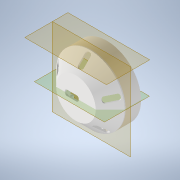
# Autodesk Inventor part: GehauseteilC
Saved by Autodesk Inventor 2020.2 (Build 242310000, 310)
## iProperties
Created: 2020-02-13
Part Number: GehauseteilC
Material: Generisch
Document SubType Name: Modeling
Designer: Max
Density: 1 g/cm^3
Appearance: Vorgabe
Author: Max
Autodesk Inventor part; units mm, degrees
ref_plane "YZ Plane" through (0, 0, 0) normal (1, 0, 0) x (0, 1, 0)
sketch "Skizze1" plane through (0, 0, 0) normal (0, 1, 0) x (-1, 0, 0)
  line L0 (0, 58.25) -> (0, 50.9382)
  line L1 (0, 85.6191) -> (0, -26.0665)
  line L2 (62.5, 0) -> (62.5, -3)
  line L3 (-64.5, 0) -> (64.5, 0) projected
  line L4 (0, 58.25) -> (-37.25, 58.25)
  line L5 (-37.25, 58.25) -> (-64.5, 31)
  line L6 (-64.5, 31) -> (-64.5, 0)
  line L7 (-64.5, 0) -> (-61.5, 0)
  line L8 (-61.5, 29.7574) -> (-36.0074, 55.25)
  line L9 (-36.0074, 55.25) -> (0, 55.25)
  line L10 (-61.5, 29.7574) -> (-61.5, 0)
  line L11 (0, 55.25) -> (0, 58.25)
  line L12 (64.5, 0) -> (-61.5, 0)
  point P0 (0, 0)
  point P1 (0, 0)
  point P2 (0, 55.25)
  dimension "d116" = 135
  dimension "d117" = 31
  dimension "d118" = 3
  dimension "d119" = 3
  dimension "d120" = 3
  dimension "d121" = 129
  dimension "d123" = 58.25
  constraints: 22 end point, 2 horizontal, 2 parallel, 2 perpendicular, 2 point on line, 1 collinear, 1 vertical, 5 other
  measures "d116" angle of L5 L6
  measures "d117" distance of L5.end L6.end
  measures "d118" distance between parallel lines of L6 L10
  measures "d119" distance between parallel lines of L5 L8
  measures "d120" distance between parallel lines of L4 L9
  measures "d121" diameter of L6 L1
  measures "d123" distance from line of point (0, 0) L4
revolve "Umdrehung1" add sketch "Skizze1" angle 360 about axis through (0, 0, 85.6191) along (0, 0, -1) contours L0 L9 L8 L10 L3 L6 L5 L4
ref_plane "Arbeitsebene12" through (0, 0, 29.125) normal (0, 0, 1) x (1, 0, 0)
ref_plane "Arbeitsebene16" through (-19.78, -4.15, 53.9382) normal (0, 0, 1) x (1, 0, 0)
ref_plane "Arbeitsebene13" through (-26.5595, -36.5552, 47.0027) normal (-0.4156269, -0.5720614, 0.7071068) x (-0.4156269, -0.5720614, -0.7071068)
sketch "Skizze26" plane through (-26.5595, -36.5552, 47.0027) normal (-0.4156269, -0.5720614, 0.7071068) x (-0.4156269, -0.5720614, -0.7071068)
  line L0 (-9, -4.15) -> (9, -4.15) projected
  line L1 (9, 4.15) -> (-9, 4.15) projected
  line L2 (12, -1.15) -> (12, 1.15) projected
  line L3 (-12, 1.15) -> (-12, -1.15) projected
  line L4 (5, -1.5) -> (5, 1.5) projected
  line L5 (5, 1.5) -> (9, 1.5) projected
  line L6 (9, 1.5) -> (9, -1.5) projected
  line L7 (9, -1.5) -> (5, -1.5) projected
  arc A0 (12, 1.15) -> (9, 4.15) centre (9, 1.15) ccw projected
  line L8 (9, 4.15) -> (-9, 4.15) projected
  arc A1 (-9, 4.15) -> (-12, 1.15) centre (-9, 1.15) ccw projected
  line L9 (-12, 1.15) -> (-12, -1.15) projected
  arc A2 (-12, -1.15) -> (-9, -4.15) centre (-9, -1.15) ccw projected
  line L10 (-9, -4.15) -> (9, -4.15) projected
  arc A3 (9, -4.15) -> (12, -1.15) centre (9, -1.15) ccw projected
  line L11 (12, -1.15) -> (12, 1.15) projected
  line L12 (14.0924, -1.5) -> (14.0924, 1.5) projected
  line L13 (14.0924, 1.5) -> (18.0924, 1.5) projected
  line L14 (18.0924, 1.5) -> (18.0924, -1.5) projected
  line L15 (18.0924, -1.5) -> (14.0924, -1.5) projected
  arc A4 (21.0924, 1.15) -> (18.0924, 4.15) centre (18.0924, 1.15) ccw projected
  line L16 (18.0924, 4.15) -> (0.0924, 4.15) projected
  arc A5 (0.0924, 4.15) -> (-2.9076, 1.15) centre (0.0924, 1.15) ccw projected
  line L17 (-2.9076, 1.15) -> (-2.9076, -1.15) projected
  arc A6 (-2.9076, -1.15) -> (0.0924, -4.15) centre (0.0924, -1.15) ccw projected
  line L18 (0.0924, -4.15) -> (18.0924, -4.15) projected
  arc A7 (18.0924, -4.15) -> (21.0924, -1.15) centre (18.0924, -1.15) ccw projected
  line L19 (21.0924, -1.15) -> (21.0924, 1.15) projected
  ellipse E0 centre (-20.635, 0.0005) end of major axis (-20.635, 64.5005) minor radius 45.6084 projected
  line L20 (0.0924, 5.15) -> (18.0924, 5.15)
  line L21 (22.0924, 1.15) -> (22.0924, -1.15)
  line L22 (18.0924, -5.15) -> (0.0924, -5.15)
  line L23 (-3.9076, -1.15) -> (-3.9076, 1.15)
  arc A8 (-3.9076, -1.15) -> (0.0924, -5.15) centre (0.0924, -1.15) ccw
  arc A9 (0.0924, 5.15) -> (-3.9076, 1.15) centre (0.0924, 1.15) ccw
  arc A10 (22.0924, 1.15) -> (18.0924, 5.15) centre (18.0924, 1.15) ccw
  arc A11 (18.0924, -5.15) -> (22.0924, -1.15) centre (18.0924, -1.15) ccw
  point P0 (1.2853, 0.0005)
  point P1 (-11.9204, -4.15)
  point P2 (12.2156, -4.15)
  point P3 (-6.7639, 0.85)
  point P4 (6.7639, 0.85)
  dimension "d124" = 1
  dimension "d125" = 1
  dimension "d126" = 1
  dimension "d127" = 1
  constraints: 10 point on circle, 8 end point, 4 centre point, 4 coincident, 4 tangent, 2 parallel, 2 point on line, 1 horizontal, 1 perpendicular, 1 other
  measures "d124" distance between parallel lines of L20 L16
  measures "d125" distance between parallel lines of L22 L18
  measures "d126" distance between parallel lines of L17 L23
  measures "d127" distance between parallel lines of L19 L21
extrude "Extrusion14" cut sketch "Skizze26" against normal mid plane 10 contours A6 L17 A5 L1 A0 L2 A3 L0 | L0 L18 A7 L19 A4 L16 L1 A9 L20 A10 L21 A11 L22 A8 | L0 A8 L23 A9 L1 A5 L17 A6 | A3 L2 A0 L16 A4 L19 A7 L18 | L4 L5 L6 L7 | L12 L13 L14 L15
ref_plane "Arbeitsebene14" through (-20.7407, -28.5463, 37.1032) normal (-0.4156269, -0.5720614, 0.7071068) x (-0.4156269, -0.5720614, -0.7071068)
ref_plane "Arbeitsebene15" through (0, 70, 0) normal (0, 1, 0) x (-1, 0, 0)
sketch "Skizze32" plane through (0, 70, 0) normal (0, 1, 0) x (-1, 0, 0)
  line L0 (-3.17, 8.66) -> (3.17, 8.66) projected
  line L1 (-3.17, 5.8) -> (3.17, 5.8) projected
  line L2 (-25.5797, 11.4942) -> (-36.763, 11.4942)
  line L3 (-36.763, 11.4942) -> (-36.763, -1.4577)
  line L4 (-36.763, -1.4577) -> (-25.5797, -1.4577)
  line L5 (-25.5797, -1.4577) -> (-25.5797, 11.4942)
  point P0 (0, 0)
  constraints: 8 end point, 2 parallel, 1 horizontal, 1 perpendicular
extrude "Kabelauslass" [suppressed]
pattern_circular "Runde Anordnung3" count 5 over 360 about axis through (0, 0, -10) along (0, 0, 1) of "Extrusion14"
ref_plane "Arbeitsebene17" through (-7.78, 0, 44.25) normal (0, 0, 1) x (0, -1, 0)
sketch "Skizze33" plane through (-7.78, 0, 44.25) normal (0, 0, 1) x (0, -1, 0)
  circle A0 centre (13.8, -12.5) radius 3
  circle A1 centre (13.8, 12.5) radius 3
  circle A2 centre (-13.8, 12.5) radius 3
  circle A3 centre (-13.8, -12.5) radius 3
  circle A4 centre (13.8, 12.5) radius 1.5 projected
  circle A5 centre (-13.8, 12.5) radius 1.5 projected
  circle A6 centre (13.8, -12.5) radius 1.5 projected
  circle A7 centre (-13.8, -12.5) radius 1.5 projected
  point P0 (0, 7.78)
  dimension "d131" = 6
  dimension "d132" = 6
  dimension "d133" = 6
  dimension "d134" = 6
  constraints: 4 centre point
  measures "d131" diameter of A1
  measures "d132" diameter of A0
  measures "d133" diameter of A3
  measures "d134" diameter of A2
extrude "Extrusion19" add sketch "Skizze33" along normal up to next
ref_plane "Arbeitsebene19" through (-41.4943, 13.4828, 32.5889) normal (-0.6724985, 0.218508, 0.7071068) x (0.309017, 0.9510565, 0)
sketch "Skizze35" plane through (-41.4943, 13.4828, 32.5889) normal (-0.6724985, 0.218508, 0.7071068) x (0.309017, 0.9510565, 0)
  circle A0 centre (13.8, -12.5) radius 1.5 projected
  circle A1 centre (13.8, 12.5) radius 1.5 projected
  circle A2 centre (-13.8, 12.5) radius 1.5 projected
  circle A3 centre (-13.8, -12.5) radius 1.5 projected
  circle A4 centre (13.8, -12.5) radius 3
  circle A5 centre (13.8, 12.5) radius 3
  circle A6 centre (-13.8, 12.5) radius 3
  circle A7 centre (-13.8, -12.5) radius 3
  point P0 (-0.0005, -7.8071)
  dimension "d143" = 6
  dimension "d144" = 6
  dimension "d145" = 6
  dimension "d146" = 6
  constraints: 4 centre point, 4 coincident
  measures "d143" diameter of A5
  measures "d144" diameter of A6
  measures "d145" diameter of A7
  measures "d146" diameter of A4
extrude "Extrusion20" add sketch "Skizze35" along normal up to next
sketch "Skizze36" plane through (-41.4943, 13.4828, 32.5889) normal (-0.6724985, 0.218508, 0.7071068) x (0.309017, 0.9510565, 0)
  line L0 (17.05, -17.5) -> (17.05, 17.5) projected
  line L1 (17.05, 17.5) -> (-17.05, 17.5) projected
  line L2 (-17.05, 17.5) -> (-17.05, -17.5) projected
  line L3 (-17.05, -17.5) -> (17.05, -17.5) projected
  line L4 (-15.55, -16) -> (-15.55, 16)
  line L5 (15.55, 16) -> (15.55, -16)
  line L6 (5.35, 17.5) -> (5.35, 16)
  line L7 (-5.35, 17.5) -> (-5.35, 16)
  line L8 (5.35, -17.5) -> (5.35, -16)
  line L9 (-5.35, -17.5) -> (-5.35, -16)
  line L10 (15.55, -16) -> (5.35, -16)
  line L11 (-5.35, -16) -> (-15.55, -16)
  line L12 (-15.55, 16) -> (-5.35, 16)
  line L13 (5.35, 16) -> (15.55, 16)
  line L14 (-17.05, -17.5) -> (-17.05, 17.5)
  line L15 (17.05, 17.5) -> (17.05, -17.5)
  line L16 (17.05, -17.5) -> (5.35, -17.5)
  line L17 (-5.35, -17.5) -> (-17.05, -17.5)
  line L18 (-17.05, 17.5) -> (-5.35, 17.5)
  line L19 (5.35, 17.5) -> (17.05, 17.5)
  point P0 (-0.0005, -7.8071)
  dimension "d147" = 1.5
  dimension "d149" = 1.5
  dimension "d151" = 10.7
  dimension "d152" = 11.7
  dimension "d153" = 10.7
  dimension "d154" = 11.7
  constraints: 32 end point, 12 perpendicular, 10 parallel, 4 horizontal, 4 point on line
  measures "d147" distance between parallel lines of L5 L0
  measures "d149" distance between parallel lines of L2 L4
  measures "d151" distance from line of L7 L6.end
  measures "d152" distance between parallel lines of L0 L6
  measures "d153" distance between parallel lines of L9 L8
  measures "d154" distance between parallel lines of L0 L8
extrude "Extrusion21" add sketch "Skizze36" along normal up to next contours L3 L8 L10 L5 L13 L6 L1 L0 | L3 L2 L1 L7 L12 L4 L11 L9
pattern_circular "Runde Anordnung4" count 5 over 360 about axis through (0, 0, 15.5) along (0, 0, -1) of "Extrusion20"
pattern_circular "Runde Anordnung5" count 5 over 360 about axis through (0, 0, 15.5) along (0, 0, -1) of "Extrusion21"
sketch "Skizze40" plane through (4.72, -13.8, 44.25) normal (0, 0, -1) x (-1, 0, 0)
  line L0 (-5, -3.25) -> (-5, 30.85) projected
  line L1 (30, -3.25) -> (-5, -3.25) projected
  line L2 (30, 30.85) -> (30, -3.25) projected
  line L3 (-5, 30.85) -> (30, 30.85) projected
  line L4 (-5, -3.25) -> (30, -3.25)
  line L5 (30, 30.85) -> (-5, 30.85)
  line L6 (-3.5, -1.75) -> (28.5, -1.75)
  line L7 (28.5, 29.35) -> (-3.5, 29.35)
  line L8 (28.5, 8.45) -> (30, 8.45)
  line L9 (28.5, 19.15) -> (30, 19.15)
  line L10 (-5, 8.45) -> (-3.5, 8.45)
  line L11 (-5, 19.15) -> (-3.5, 19.15)
  line L12 (-5, 30.85) -> (-5, 19.15)
  line L13 (-5, 8.45) -> (-5, -3.25)
  line L14 (-3.5, 29.35) -> (-3.5, 19.15)
  line L15 (-3.5, 8.45) -> (-3.5, -1.75)
  line L16 (28.5, -1.75) -> (28.5, 8.45)
  line L17 (28.5, 19.15) -> (28.5, 29.35)
  line L18 (30, -3.25) -> (30, 8.45)
  line L19 (30, 19.15) -> (30, 30.85)
  point P0 (4.72, 13.8)
  point P1 (30, 19.15)
  point P2 (-5, 19.15)
  dimension "d182" = 1.5
  dimension "d184" = 1.5
  dimension "d185" = 10.7
  dimension "d186" = 11.7
  dimension "d187" = 10.7
  dimension "d188" = 11.7
  constraints: 32 end point, 11 perpendicular, 10 parallel, 2 horizontal
  measures "d182" distance between parallel lines of L3 L7
  measures "d184" distance between parallel lines of L6 L1
  measures "d185" distance between parallel lines of L11 L10
  measures "d186" distance between parallel lines of L3 L11
  measures "d187" distance between parallel lines of L9 L8
  measures "d188" distance between parallel lines of L3 L9
extrude "Extrusion25" add sketch "Skizze40" against normal up to next contours L0 L10 L15 L6 L16 L8 L2 L1 | L0 L3 L2 L9 L17 L7 L14 L11
sketch "Skizze41" plane through (-7.78, 0, 44.25) normal (0, 0, -1) x (-1, 0, 0)
  line L0 (-17.5, -5.35) -> (-17.5, -17.05) projected
  line L1 (-17.5, 5.35) -> (-16, 5.35) projected
  line L2 (-17.5, -5.35) -> (-16, -5.35)
  line L3 (-16, -5.35) -> (-16, 5.35)
  line L4 (-16, 5.35) -> (-17.5, 5.35)
  line L5 (-17.5, 5.35) -> (-17.5, -5.35)
  line L6 (17.5, 17.05) -> (17.5, 5.35) projected
  line L7 (16, -5.35) -> (17.5, -5.35)
  line L8 (17.5, -5.35) -> (17.5, 5.35)
  line L9 (17.5, 5.35) -> (16, 5.35)
  line L10 (16, 5.35) -> (16, -5.35)
  point P0 (-7.78, 0)
  constraints: 16 end point, 4 parallel, 2 horizontal, 2 perpendicular
ref_plane "Arbeitsebene22" through (0.72, -5.3, 50.45) normal (0, 0, 1) x (1, 0, 0)
extrude "Extrusion26" add sketch "Skizze41" against normal up to surface (4.8 mm away) from surface at -6.2
sketch "Skizze42" plane through (-5.3495, 31.2555, 44.9633) normal (0, -0.7071068, -0.7071068) x (-1, 0, 0)
  line L0 (-10.7, 35) -> (-10.7, 33.5) projected
  line L1 (0, 35) -> (11.7, 35) projected
  line L2 (-10.7, 33.5) -> (0, 33.5)
  line L3 (0, 33.5) -> (0, 35)
  line L4 (0, 35) -> (-10.7, 35)
  line L5 (-10.7, 35) -> (-10.7, 33.5)
  point P0 (-5.3495, 9.6929)
  point P1 (-10.7, 35)
  constraints: 8 end point, 2 parallel, 1 horizontal, 1 perpendicular
ref_plane "Arbeitsebene23" through (-5.2995, 57.2063, 27.7806) normal (0, 0.7071068, 0.7071068) x (0, -0.7071068, 0.7071068)
extrude "Extrusion27" add sketch "Skizze42" against normal up to surface from surface at -6.2 round surface about axis through (0, 0, 14.8787) along (0, 0, -1) radius 61.5 far side no
sketch "Skizze43" plane through (17.0505, 56.0042, 20.2146) normal (0, -0.7071068, -0.7071068) x (-1, 0, 0)
  line L0 (1.5, -33.5) -> (11.7, -33.5) projected
  line L1 (34.1, -35) -> (22.4, -35) projected
  line L2 (11.7, -33.5) -> (22.4, -33.5)
  line L3 (22.4, -33.5) -> (22.4, -35)
  line L4 (22.4, -35) -> (11.7, -35)
  line L5 (11.7, -35) -> (11.7, -33.5)
  point P0 (17.0505, -25.3071)
  constraints: 8 end point, 2 parallel, 1 horizontal, 1 perpendicular
ref_plane "Arbeitsebene24" through (-5.2995, 38.8215, 46.1654) normal (0, 0.7071068, 0.7071068) x (0, -0.7071068, 0.7071068)
extrude "Extrusion28" add sketch "Skizze43" against normal up to surface from surface at -6.2 round surface about axis through (0, 0, 42.5037) along (0, 0, -1) radius 48.7537 half angle 45 far side no
pattern_circular "Runde Anordnung6" count 5 over 360 about axis through (0, 0, 15.5) along (0, 0, -1) of "Extrusion27"
pattern_circular "Runde Anordnung7" count 5 over 360 about axis through (0, 0, 15.5) along (0, 0, -1) of "Extrusion28"
sketch "Skizze44" plane through (0, 0, 58.25) normal (0, 0, 1) x (1, 0, 0)
  line L0 (-2.78, -1.5) -> (-2.78, 1.5) projected
  line L1 (-2.78, 1.5) -> (1.22, 1.5) projected
  line L2 (1.22, 1.5) -> (1.22, -1.5) projected
  line L3 (1.22, -1.5) -> (-2.78, -1.5) projected
  arc A0 (4.22, 1.15) -> (1.22, 4.15) centre (1.22, 1.15) ccw projected
  line L4 (1.22, 4.15) -> (-16.78, 4.15) projected
  arc A1 (-16.78, 4.15) -> (-19.78, 1.15) centre (-16.78, 1.15) ccw projected
  line L5 (-19.78, 1.15) -> (-19.78, -1.15) projected
  arc A2 (-19.78, -1.15) -> (-16.78, -4.15) centre (-16.78, -1.15) ccw projected
  line L6 (-16.78, -4.15) -> (1.22, -4.15) projected
  arc A3 (1.22, -4.15) -> (4.22, -1.15) centre (1.22, -1.15) ccw projected
  line L7 (4.22, -1.15) -> (4.22, 1.15) projected
  line L8 (1.22, -5.15) -> (-16.78, -5.15)
  line L9 (-20.78, -1.15) -> (-20.78, 1.15)
  line L10 (-16.78, 5.15) -> (1.22, 5.15)
  line L11 (5.22, 1.15) -> (5.22, -1.15)
  arc A4 (-16.78, 5.15) -> (-20.78, 1.15) centre (-16.78, 1.15) ccw
  arc A5 (-20.78, -1.15) -> (-16.78, -5.15) centre (-16.78, -1.15) ccw
  arc A6 (1.22, -5.15) -> (5.22, -1.15) centre (1.22, -1.15) ccw
  arc A7 (5.22, 1.15) -> (1.22, 5.15) centre (1.22, 1.15) ccw
  point P0 (0, 0)
  dimension "d203" = 1
  dimension "d204" = 1
  dimension "d205" = 1
  dimension "d206" = 1
  constraints: 14 point on circle, 8 end point, 4 centre point, 4 coincident, 4 tangent, 2 parallel, 1 horizontal, 1 perpendicular
  measures "d203" distance between parallel lines of L8 L6
  measures "d204" distance between parallel lines of L4 L10
  measures "d205" distance between parallel lines of L9 L5
  measures "d206" distance between parallel lines of L11 L7
extrude "Extrusion29" cut sketch "Skizze44" against normal up to surface (3 mm away) contours L0 L1 L2 L3 | L7 A3 L6 A2 L5 A1 L4 A0 | L8 A5 L9 A4 L10 A7 L11 A6
fillet "Rundung1" radius 0.3 48 edges at (44.0662, 9.9104, 50.3331) (41.9209, 13.6204, 51.4219) (41.4758, 17.8828, 50.3333) (48.5899, 21.2024, 42.4857) (57.0992, 22.9599, 33.9576) (59.4058, 19.3016, 33.0371) (59.6889, 14.9837, 33.9591) (51.7727, 11.4065, 42.4856) (23.0426, -38.8469, 50.3332) (25.9081, -35.6602, 51.4219) (29.8243, -33.9197, 50.3333) (35.1797, -39.6598, 42.4857) (39.4814, -47.2069, 33.9591) (36.7144, -50.5338, 33.0371) (32.6953, -52.1373, 33.9591) (26.8468, -45.714, 42.4856) (-32.6987, -52.137, 33.9576) (-36.7151, -50.5332, 33.0371) (-39.4821, -47.2064, 33.9591) (-35.1805, -39.6593, 42.4856) (-29.825, -33.9191, 50.3332) (-25.9088, -35.6596, 51.4219) (-23.0434, -38.8463, 50.3333) (-26.8476, -45.7135, 42.4857) (4.1918, 44.9719, 50.3331) (0.0005, 44.0781, 51.4219) (-4.1908, 44.9719, 50.3333) (-5.1495, 52.7636, 42.4857) (-4.1936, 61.3978, 33.9591) (0.0005, 62.4629, 33.0371) (4.1945, 61.3978, 33.9591) (5.1505, 52.7636, 42.4856) (-59.6897, 14.9871, 33.9576) (-59.4056, 19.3025, 33.0371) (-57.0966, 22.9622, 33.9591) (-48.5896, 21.2032, 42.4856) (-41.4754, 17.8837, 50.3332) (-41.9206, 13.6213, 51.4219) (-44.0659, 9.9114, 50.3333) (-51.7725, 11.4074, 42.4857) (-19.6084, -3.9784, 58.25) (-20.78, 0, 58.25) (-19.6084, 3.9784, 58.25) (-7.78, 5.15, 58.25) (4.0484, 3.9784, 58.25) (5.22, 0, 58.25) (4.0484, -3.9784, 58.25) (-7.78, -5.15, 58.25)
ref_plane "Arbeitsebene25" through (-1.5625, -0.0003, 0.5181) normal (0, -1, 0) x (1, 0, 0)
sketch "Skizze45" plane through (-1.5625, -0.0003, 0.5181) normal (0, -1, 0) x (1, 0, 0)
  line L0 (66.0625, 30.4819) -> (66.0625, -0.5181) projected
  line L1 (-62.9375, -0.5181) -> (66.0625, -0.5181) projected
  line L2 (63.0625, -0.5181) -> (60.0625, -0.5181)
  line L3 (63.0625, 2.4819) -> (63.0625, -0.5181)
  line L4 (60.0625, -0.5181) -> (63.0625, 2.4819)
  line L5 (1.5625, -6.7181) -> (1.5625, 36.6819) projected
  point P0 (1.5625, -0.5181)
  dimension "d210" = 3
  dimension "d212" = 3
  dimension "d213" = 3
  constraints: 6 end point, 1 horizontal, 1 point on line
  measures "d210" distance between parallel lines of L0 L3
  measures "d212" distance of L2.start L2.end
  measures "d213" distance of L3.start L2.start
revolve "Umdrehung2" add sketch "Skizze45" angle 360 about axis through (0, -0.0003, -10) along (0, 0, 1)
sketch "Skizze48" plane through (0, 0, 0) normal (0, 0, -1) x (-1, 0, 0)
  circle A0 centre (0, -0.0003) radius 58.5 projected
  circle A1 centre (0, 0) radius 61.5 projected
  line L0 (-55.965, 15.2279) -> (-56.4476, 15.3592)
  line L1 (23.2493, -53.1363) -> (24.6523, -56.3428)
  line L2 (-11.4326, -56.8596) -> (-12.123, -60.2933)
  line L3 (-56.8617, 11.433) -> (-60.2933, 12.123)
  line L4 (-53.1341, -23.2483) -> (-56.3428, -24.6523)
  line L5 (53.1361, 23.2492) -> (56.3428, 24.6523)
  line L6 (56.862, -11.433) -> (60.2933, -12.123)
  line L7 (11.5315, 57.3519) -> (12.123, 60.2933)
  line L8 (-23.4496, 53.5941) -> (-24.6523, 56.3428)
  arc A2 (53.1361, 23.2492) -> (11.433, 56.8617) centre (0, 0) ccw
  arc A3 (56.3428, 24.6523) -> (12.123, 60.2933) centre (0, 0) ccw
  arc A4 (23.2493, -53.1363) -> (56.862, -11.433) centre (0, 0) ccw
  arc A5 (24.6523, -56.3428) -> (60.2933, -12.123) centre (0, 0) ccw
  arc A6 (-23.2492, 53.1361) -> (-56.8617, 11.433) centre (0, 0) ccw
  arc A7 (-53.1341, -23.2483) -> (-11.4326, -56.8596) centre (0, 0) ccw
  arc A8 (-24.6523, 56.3428) -> (-60.2933, 12.123) centre (0, 0) ccw
  arc A9 (-56.3428, -24.6523) -> (-12.123, -60.2933) centre (0, 0) ccw
  point P0 (0, 0)
  point P1 (-36.2179, 45.9401)
  point P2 (-57.3521, 11.5316)
  point P3 (36.2179, 45.9401)
  point P4 (53.5943, 23.4497)
  point P5 (57.3522, -11.5316)
  point P6 (23.4498, -53.5947)
  dimension "d236" = 35
  dimension "d237" = 55
  dimension "d238" = 35
  dimension "d239" = 55
  dimension "d240" = 35
  dimension "d241" = 55
  dimension "d242" = 35
  dimension "d243" = 55
  dimension "d246" = 3.5025
  dimension "d247" = 3.5002
  dimension "d248" = 3.5002
  dimension "d249" = 3.5
  constraints: 20 point on circle, 18 end point, 8 centre point, 2 coincident, 2 point on line
  measures "d236" angle of L5 L6
  measures "d237" angle of L1 L6
  measures "d238" angle of L2 L1
  measures "d239" angle of L2 L4
  measures "d240" angle of L3 L4
  measures "d241" angle of L7 L5
  measures "d242" angle of L7 L8
  measures "d243" angle of L8 L3
  measures "d246" radial gap between concentric circles of A1 A7
  measures "d247" radial gap between concentric circles of A1 A6
  measures "d248" radial gap between concentric circles of A2 A1
  measures "d249" radial gap between concentric circles of A1 A4
extrude "Extrusion30" cut sketch "Skizze48" against normal blind 10 contours L7 A1 L5 A0 | A0 L3 A1 L8 | L6 A1 L1 A0 | L4 A7 L2 A0 | A0 L2 A1 L4
